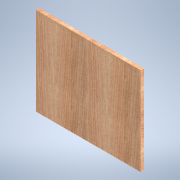
# Autodesk Inventor part: Boden
Saved by Autodesk Inventor 2021 (Build 250183000, 183)
## iProperties
Created: 2022-06-26
Part Number: Boden
Material: Holz (Birke)
Document SubType Name: Modeling
Designer: adria
Density: 0.55 g/cm^3
Appearance: Birke - natur - poliert
Mass: 1847.75 g
Surface Area: 4499.87 cm^2
Volume: 3359.55 cm^3
Author: adria
Autodesk Inventor part; units mm, degrees
ref_plane "YZ Plane" through (0, 0, 0) normal (1, 0, 0) x (0, 1, 0)
ref_plane "XZ Plane" through (0, 0, 0) normal (0, 1, 0) x (-1, 0, 0)
ref_plane "XY Plane" through (0, 0, 0) normal (0, 0, 1) x (1, 0, 0)
sketch "Skizze1" plane through (0, 0, 0) normal (0, 0, 1) x (1, 0, 0)
  line L0 (-250, -210) -> (250, -210)
  line L1 (250, -210) -> (250, 210)
  line L2 (250, 210) -> (-250, 210)
  line L3 (-250, 210) -> (-250, -210)
  line L4 (-250, -210) -> (250, 210) construction
  line L5 (250, -210) -> (-250, 210) construction
  point P0 (0, 0)
  dimension "d0" = 500
  dimension "d1" = 420
  constraints: 12 end point, 2 midpoint, 2 parallel, 1 horizontal, 1 perpendicular
  measures "d0" distance of L2.end L1.end
  measures "d1" distance of L1.end L0.end
extrude "Extrusion1" add sketch "Skizze1" along normal blind 16
sketch "Skizze3" plane through (0, 0, 16) normal (0, 0, 1) x (1, 0, 0)
  line L0 (0, -294) -> (0, 294) projected
  line L1 (-350, 0) -> (350, 0) projected
  line L2 (-250, 210) -> (-250, -210) projected
  point P0 (0, 0)
  point P1 (8.3767, 8.3767)
  point P2 (-8.3767, 8.3767)
  point P3 (-8.3767, -8.3767)
  point P4 (8.3767, -8.3767)
  point P5 (-15.5, 15.5)
  point P6 (15.5, 15.5)
  point P7 (-15.5, -15.5)
  point P8 (15.5, -15.5)
  dimension "d15" = 360
  dimension "d39" = 31
  dimension "d40" = 31
  dimension "d41" = 234.5
  constraints: 2 horizontal alignment, 2 vertical alignment, 1 symmetric about line, 5 other
  measures "d39" distance of point (-15.5, 15.5) point (15.5, 15.5)
  measures "d40" distance of point (15.5, -15.5) point (15.5, 15.5)
  measures "d41" distance from line of L2 point (-15.5, 15.5)
hole "Bohrung2" at (-15.5, 15.5, 16) at (15.5, 15.5, 16) at (15.5, -15.5, 16) at (-15.5, -15.5, 16) direction (0, 0, -1) diameter 3 end through all
equation "\"d40\" = d39"
